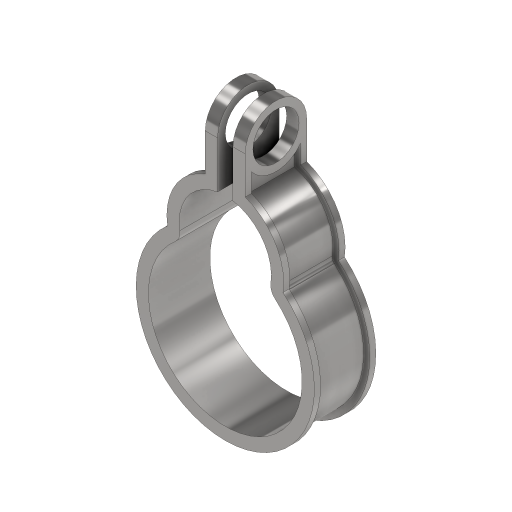
# Autodesk Inventor part: Part015. Double clip
Saved by Autodesk Inventor 2023.2 (Build 272271030, 271C)
## iProperties
Created: 2023-09-19
Part Number: Part015. Double clip
Material: Steel, Carbon
Document SubType Name: Modeling
Designer: User
Mass: 82.56 g
Surface Area: 115.492 cm^2
Volume: 10.5172 cm^3
Density: 7.85 g/cm^3
Appearance: Steel - Polished
Author: User
Autodesk Inventor part; units mm, degrees
ref_plane "XZ Plane" through (0, 0, 0) normal (0, 1, 0) x (-1, 0, 0)
ref_plane "XY Plane" through (0, 0, 0) normal (0, 0, 1) x (1, 0, 0)
sketch "Sketch1" plane through (0, 0, 0) normal (0, 0, 1) x (1, 0, 0)
  arc A0 (-16.1874, 19.0517) -> (16.1874, 19.0517) centre (0, 0) ccw
  line L0 (-2.5, 50.7018) -> (-2.5, 39.7902) construction
  line L1 (2.5, 50.7018) -> (2.5, 39.7902) construction
  line L2 (2.5, 50.7018) -> (-2.5, 50.7018) construction
  arc A1 (14.8242, 22.7105) -> (2.5, 39.7902) centre (0, 25) ccw
  arc A2 (-2.5, 39.7902) -> (-14.8242, 22.7105) centre (0, 25) ccw
  arc A3 (-16.1874, 19.0517) -> (-14.8242, 22.7105) centre (-18.7774, 22.1) ccw
  arc A4 (14.8242, 22.7105) -> (16.1874, 19.0517) centre (18.7774, 22.1) ccw
  dimension "d0" = 25
  dimension "d2" = 25
  dimension "d3" = 5
  dimension "d4" = 4
  constraints: 10 point on circle, 6 end point, 5 centre point, 4 tangent, 2 parallel, 1 coincident, 1 equal radius, 1 perpendicular, 1 vertical, 1 vertical alignment
  measures "d0" radius of A0
  measures "d2" distance of point (0, 0) A1.centre
  measures "d3" distance between parallel lines of L1 L0
  measures "d4" radius of A3
sketch "Sketch2" plane through (0, 0, 0) normal (1, 0, 0) x (0, 1, 0)
  line L0 (-25, 10) -> (-25, -10)
  line L1 (-25, -10) -> (-29, -10)
  line L2 (-29, -10) -> (-29, -8)
  line L3 (-29, -8) -> (-27, -8)
  line L4 (-27, -8) -> (-27, 8)
  line L5 (-27, 8) -> (-29, 8)
  line L6 (-29, 8) -> (-29, 10)
  line L7 (-29, 10) -> (-25, 10)
  line L8 (19.0517, 0) -> (-25, 0) projected
  point P0 (0, 0)
  point P1 (19.0517, 0)
  dimension "d5" = 20
  dimension "d6" = 2
  dimension "d8" = 4
  dimension "d9" = 2
  constraints: 16 end point, 6 perpendicular, 2 equal length, 2 point on line, 1 midpoint, 1 vertical
  measures "d5" distance of L0.start L0.end
  measures "d6" distance of L5.end L6.end
  measures "d8" distance of L6.end L0.start
  measures "d9" distance between parallel lines of L4 L0
sweep "Sweep1" add profiles "Sketch2" path "Sketch1"
ref_plane "Work Plane1" through (-2.5, 39.7902, 10) normal (1, 0, 0) x (0, 1, 0)
sketch "Sketch3" plane through (-2.5, 39.7902, 10) normal (1, 0, 0) x (0, 1, 0)
  line L0 (0, 0) -> (0, -20)
  line L1 (0, -20) -> (15.2098, -20)
  arc A0 (15.2098, -20) -> (15.2098, 0) centre (15.2098, -10) ccw
  line L2 (15.2098, 0) -> (0, 0)
  line L3 (3.9441, 0) -> (3.9441, -2) projected
  point P0 (-39.7902, -10)
  dimension "d12" = 55
  constraints: 6 end point, 2 point on circle, 2 tangent, 1 centre point, 1 horizontal, 1 perpendicular, 1 vertical
  measures "d12" distance of point (-39.79, -10) A0.centre
extrude "Extrusion1" add sketch "Sketch3" against normal blind 2
sketch "Sketch4" plane through (-4.5, 39.7902, 10) normal (-1, 0, 0) x (0, 0, 1)
  line L0 (-2, 3.6692) -> (-2, 1.6034) construction
  line L1 (0, 3.6692) -> (0, 15.2098) projected
  arc A0 (0, 15.2098) -> (-20, 15.2098) centre (-10, 15.2098) ccw projected
  line L2 (-20, 15.2098) -> (-20, 3.6692) projected
  arc A1 (-18, 9.2098) -> (-2, 9.2098) centre (-10, 15.2098) ccw
  line L3 (-20, 3.6692) -> (-20, 1.6034)
  line L4 (-20, 3.9441) -> (-20, 0) projected
  line L5 (-18, 1.6034) -> (-18, 9.2098)
  line L6 (-18, 1.972) -> (-18, 3.9441) projected
  line L7 (-18, 1.6034) -> (-20, 1.6034)
  line L8 (0, 3.6692) -> (0, 1.6034)
  line L9 (0, -17.6902) -> (0, 3.9441) projected
  line L10 (0, 1.6034) -> (-2, 1.6034)
  line L11 (-2, 1.6034) -> (-2, 9.2098)
  point P0 (-10, -39.7902)
  constraints: 13 end point, 3 point on line, 2 point on circle, 1 centre point, 1 coincident, 1 collinear, 1 concentric, 1 horizontal, 1 perpendicular
extrude "Extrusion2" add sketch "Sketch4" along normal blind 2
mirror "Mirror1" about plane through (0, 0, 0) normal (1, 0, 0) of "Extrusion1", "Extrusion2"
sketch "Sketch5" plane through (-6.5, 39.7902, 10) normal (-1, 0, 0) x (0, 0, 1)
  arc A0 (0, 15.2098) -> (-20, 15.2098) centre (-10, 15.2098) ccw projected
  point P0 (-10, -39.7902)
  constraints: 1 coincident
hole "Hole1" at (-6.5, 55, 0) direction (1, 0, 0) diameter 15 end through all
body "Solid1"
